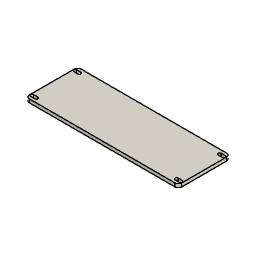
Upper Level Mount - Blank (Autodesk Fusion 360 design; units mm, degrees)
Autodesk Fusion 360 part; units mm, degrees
sketch "Sketch1" plane through (0, 0, 0) normal (0, 0, 1) x (-1, 0, 0)
  line L0 (-88.5, 30) -> (88.5, 30)
  line L1 (88.5, 30) -> (88.5, -30)
  line L2 (88.5, -30) -> (-88.5, -30)
  line L3 (-88.5, -30) -> (-88.5, 30)
  point P0 (0, 30)
  point P1 (-88.5, 0)
  dimension "d44_2_2" = 177
  dimension "d45_2_2" = 60
  dimension "d54_2_2" = 30
  dimension "d55_2_2" = 87.5
  constraint horizontal L0
  constraint vertical L1
  constraint horizontal L2
  constraint vertical L3
  constraint midpoint L0 P0
  constraint midpoint L3 P1
  constraint vertical origin P0
  constraint horizontal origin P1
  measures "d44_2_2" distance of L0.start L0.end
  measures "d45_2_2" distance of L0.start L2.end
  measures "d54_2_2" distance of L0.start P1
extrude "Extrude1" add sketch "Sketch1" along normal blind 4
fillet "Fillet1" radius 4 4 edges at (88.5, 30, 2) (88.5, -30, 2) (-88.5, 30, 2) (-88.5, -30, 2)
sketch "Sketch3" plane through (0, 0, 4) normal (0, 0, 1) x (-1, 0, 0)
  arc A0 (88.5, 26) -> (84.5, 30) centre (84.5, 26) ccw
  line L0 (84.5, 30) -> (-84.5, 30)
  arc A1 (-84.5, 30) -> (-88.5, 26) centre (-84.5, 26) ccw
  line L1 (-88.5, 26) -> (-88.5, -26)
  arc A2 (-88.5, -26) -> (-84.5, -30) centre (-84.5, -26) ccw
  line L2 (-84.5, -30) -> (84.5, -30)
  arc A3 (84.5, -30) -> (88.5, -26) centre (84.5, -26) ccw
  line L3 (88.5, -26) -> (88.5, 26)
  line L4 (0, -30) -> (0, -24.8801)
  line L5 (0, -24.8801) -> (0, 30) construction
  circle A4 centre (86.5, -25) radius 1.7
  circle A5 centre (86.5, 25) radius 1.7
  circle A6 centre (-86.5, -25) radius 1.7
  circle A7 centre (-86.5, 25) radius 1.7
  line L6 (86.5, -23.3) -> (81.5, -23.3)
  arc A8 (81.5, -23.3) -> (81.5, -26.7) centre (81.5, -25) ccw
  line L7 (81.5, -26.7) -> (86.5, -26.7)
  arc A9 (86.5, -26.7) -> (86.5, -23.3) centre (86.5, -25) ccw
  line L8 (86.5, -25) -> (81.5, -25) construction
  line L9 (86.5, 26.7) -> (81.5, 26.7)
  arc A10 (81.5, 26.7) -> (81.5, 23.3) centre (81.5, 25) ccw
  line L10 (81.5, 23.3) -> (86.5, 23.3)
  arc A11 (86.5, 23.3) -> (86.5, 26.7) centre (86.5, 25) ccw
  line L11 (86.5, 25) -> (81.5, 25) construction
  line L12 (-86.5, -26.7) -> (-81.5, -26.7)
  arc A12 (-81.5, -26.7) -> (-81.5, -23.3) centre (-81.5, -25) ccw
  line L13 (-81.5, -23.3) -> (-86.5, -23.3)
  arc A13 (-86.5, -23.3) -> (-86.5, -26.7) centre (-86.5, -25) ccw
  line L14 (-86.5, -25) -> (-81.5, -25) construction
  line L15 (-86.5, 23.3) -> (-81.5, 23.3)
  arc A14 (-81.5, 23.3) -> (-81.5, 26.7) centre (-81.5, 25) ccw
  line L16 (-81.5, 26.7) -> (-86.5, 26.7)
  arc A15 (-86.5, 26.7) -> (-86.5, 23.3) centre (-86.5, 25) ccw
  line L17 (-86.5, 25) -> (-81.5, 25) construction
  dimension "d56_2_2" = 3.4
  dimension "d57_2_2" = 3.4
  dimension "d58_2_2" = 3.4
  dimension "d59_2_2" = 3.4
  dimension "d61_2_2" = 5
  dimension "d6" = 171
  dimension "d7" = 3.4
  dimension "d8" = 5
  dimension "d9" = 3.4
  dimension "d10" = 3.4
  dimension "d11" = 3.4
  dimension "d12" = 5
  dimension "d13" = 50
  constraint midpoint L2 L4.start
  constraint midpoint L0 L5.end
  constraint horizontal A4.centre A6.centre
  constraint vertical A6.centre A7.centre
  constraint horizontal A5.centre A7.centre
  constraint vertical A4.centre A5.centre
  constraint symmetric L5 A4.centre A6.centre
  constraint tangent L6 A8
  constraint tangent A8 L7
  constraint parallel L6 L7
  constraint tangent L7 A9
  constraint tangent L6 A9
  constraint parallel L2 L8
  constraint coincident A4.centre A9.centre
  constraint tangent L9 A10
  constraint tangent A10 L10
  constraint parallel L9 L10
  constraint tangent L10 A11
  constraint tangent L9 A11
  constraint horizontal L11
  constraint coincident A5.centre A11.centre
  constraint tangent L12 A12
  constraint tangent A12 L13
  constraint parallel L12 L13
  constraint tangent L13 A13
  constraint tangent L12 A13
  constraint horizontal L14
  constraint coincident A6.centre A13.centre
  constraint tangent L15 A14
  constraint tangent A14 L16
  constraint parallel L15 L16
  constraint tangent L16 A15
  constraint tangent L15 A15
  constraint horizontal L17
  constraint coincident A7.centre A15.centre
  constraint vertical A8.centre A10.centre
  constraint vertical A12.centre A14.centre
  measures "d56_2_2" diameter of A4
  measures "d57_2_2" diameter of A6
  measures "d58_2_2" diameter of A5
  measures "d59_2_2" diameter of A7
  measures "d61_2_2" distance of L2 A4.centre
  measures "d6" horizontal distance of A2.centre A4.centre
  measures "d7" diameter of A8
  measures "d8" distance of A4.centre A8.centre
  measures "d9" diameter of A10
  measures "d10" diameter of A12
  measures "d11" diameter of A14
  measures "d12" distance of A6.centre A12.centre
  measures "d13" distance of A4.centre A5.centre
extrude "Extrude3" cut sketch "Sketch3" against normal through all contours A4 A9 | A4 L6 A8 L7 | A5 A11 | A5 L9 A10 L10 | A6 A13 | A6 L12 A12 L13 | A7 A15 | A7 L15 A14 L16
equation "d57_2_2 = d56_2_2"
equation "d58_2_2 = d56_2_2"
equation "d59_2_2 = d56_2_2"
